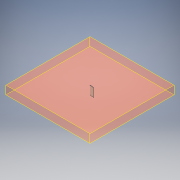
# Autodesk Inventor part: NACA63-010
Saved by Autodesk Inventor 2018 (Build 220112000, 112)
## iProperties
Created: 2019-05-16
Part Number: NACA63-010
Material: 一般
Document SubType Name: Modeling
Designer: Fluidlab
Density: 1 g/cm^3
Appearance: 既定
Author: Fluidlab
Autodesk Inventor part; units mm, degrees
ref_plane "YZ Plane" through (0, 0, 0) normal (1, 0, 0) x (0, 1, 0)
ref_plane "XZ Plane" through (0, 0, 0) normal (0, 1, 0) x (-1, 0, 0)
ref_plane "XY Plane" through (0, 0, 0) normal (0, 0, 1) x (1, 0, 0)
sketch "スケッチ1" plane through (0, 0, 0) normal (0, 0, 1) x (1, 0, 0)
  spline S0 degree 4 poles (1, -0.0002) (0.9687, -0.0034) (0.925, -0.0078) (0.8688, -0.0135) (0.8, -0.0204) (0.75, -0.0255) (0.7, -0.0305) (0.65, -0.0353) (0.6, -0.0395) (0.55, -0.0432) (0.5, -0.0463) (0.45, -0.0486) (0.4, -0.0499) (0.3501, -0.0502) (0.2998, -0.0494) (0.2504, -0.0474) (0.1997, -0.0442) (0.1565, -0.0406) (0.1024, -0.034) (0.0784, -0.0298) (0.0536, -0.0255) (0.0288, -0.0186) (0.0155, -0.0145) (0.007, -0.0094) (0.0056, -0.0091) (-0.0036, 0) (0.0056, 0.0091) (0.007, 0.0094) (0.0155, 0.0145) (0.0288, 0.0186) (0.0536, 0.0255) (0.0784, 0.0298) (0.1024, 0.034) (0.1565, 0.0406) (0.1997, 0.0442) (0.2504, 0.0474) (0.2998, 0.0494) (0.3501, 0.0502) (0.4, 0.0499) (0.45, 0.0486) (0.5, 0.0463) (0.55, 0.0432) (0.6, 0.0395) (0.65, 0.0353) (0.7, 0.0305) (0.75, 0.0255) (0.8, 0.0204) (0.8688, 0.0135) (0.925, 0.0078) (0.9687, 0.0034) (1, 0.0002) knots 0 0 0 0 0 0.057717 0.080803 0.10389 0.126974 0.150054 0.173128 0.196192 0.219247 0.242292 0.265329 0.288362 0.311394 0.33443 0.357479 0.380549 0.401957 0.421715 0.439846 0.455181 0.468356 0.478831 0.487682 0.49607 0.50393 0.512318 0.521169 0.531644 0.544819 0.560154 0.578285 0.598043 0.619451 0.642521 0.66557 0.688606 0.711638 0.734671 0.757708 0.780753 0.803808 0.826872 0.849946 0.873026 0.89611 0.919197 0.942283 1 1 1 1 1
  line L0 (1, 0.0002) -> (1, -0.0002)
  point P0 (0.95, -0.0053)
  point P1 (0.9, -0.0103)
  point P2 (0.85, -0.0154)
  point P3 (0.8, -0.0204)
  point P4 (0.75, -0.0255)
  point P5 (0.7, -0.0304)
  point P6 (0.65, -0.0352)
  point P7 (0.6, -0.0394)
  point P8 (0.55, -0.0431)
  point P9 (0.5, -0.0461)
  point P10 (0.45, -0.0484)
  point P11 (0.4, -0.0497)
  point P12 (0.35, -0.05)
  point P13 (0.3, -0.0491)
  point P14 (0.25, -0.0471)
  point P15 (0.2, -0.044)
  point P16 (0.15, -0.0395)
  point P17 (0.1, -0.0332)
  point P18 (0.075, -0.0292)
  point P19 (0.05, -0.0241)
  point P20 (0.025, -0.0174)
  point P21 (0.0125, -0.0125)
  point P22 (0.0075, -0.0098)
  point P23 (0.005, -0.0082)
  point P24 (0, 0)
  point P25 (0.005, 0.0082)
  point P26 (0.0075, 0.0098)
  point P27 (0.0125, 0.0125)
  point P28 (0.025, 0.0174)
  point P29 (0.05, 0.0241)
  point P30 (0.075, 0.0292)
  point P31 (0.1, 0.0332)
  point P32 (0.15, 0.0395)
  point P33 (0.2, 0.044)
  point P34 (0.25, 0.0471)
  point P35 (0.3, 0.0491)
  point P36 (0.35, 0.05)
  point P37 (0.4, 0.0497)
  point P38 (0.45, 0.0484)
  point P39 (0.5, 0.0461)
  point P40 (0.55, 0.0431)
  point P41 (0.6, 0.0394)
  point P42 (0.65, 0.0352)
  point P43 (0.7, 0.0304)
  point P44 (0.75, 0.0255)
  point P45 (0.8, 0.0204)
  point P46 (0.85, 0.0154)
  point P47 (0.9, 0.0103)
  point P48 (0.95, 0.0053)
  constraints: 2 end point, 1 vertical, 51 other
extrude "押し出し1" add sketch "スケッチ1" along normal blind 2
sketch "スケッチ2" plane through (0, 0, 2) normal (0, 0, 1) x (1, 0, 0)
  line L0 (-10, 10) -> (10, 10)
  line L1 (10, 10) -> (10, -10)
  line L2 (10, -10) -> (-10, -10)
  line L3 (-10, -10) -> (-10, 10)
  point P0 (0, 0)
  dimension "d2" = 20
  dimension "d3" = 20
  dimension "d5" = 10
  dimension "d12" = 10
  constraints: 8 end point, 2 parallel, 1 horizontal, 1 perpendicular
  measures "d2" distance of L0.end L1.end
  measures "d3" distance of L1.end L2.end
  measures "d5" distance from line of L0 point (0, 0)
  measures "d12" distance from line of L3 point (0, 0)
surface extrude "押し出しサーフェス1" sketch "スケッチ2" against normal blind 2 shown yes curves L0 L1 L2 L3
sketch "スケッチ3" plane through (-10, 10, 2) normal (0, 1, 0) x (1, 0, 0)
  line L0 (0, 0) -> (20, 0) projected
  line L1 (0, 2) -> (20, 2) projected
  point P0 (10, 2)
surface extrude "押し出しサーフェス2" sketch "スケッチ3" against normal up to surface (20 mm away) shown yes curves L1
sketch "スケッチ4" plane through (-10, 10, 2) normal (0, 1, 0) x (1, 0, 0)
  line L0 (0, 0) -> (20, 0) projected
  point P0 (10, 2)
surface extrude "押し出しサーフェス3" sketch "スケッチ4" against normal up to surface (20 mm away) shown yes curves L0
move or copy body "ボディを移動1" bodies to move or copy 1 copy no rotation origin (0, 0, 0) rotation axis (0, 0, 1) rotation angle -5
body "Srf1"
body "Srf2"
body "Srf3"
